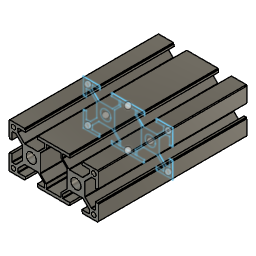
Aluminium extrusion 6030 v2 (Autodesk Fusion 360 design; units mm, degrees)
Autodesk Fusion 360 part; units mm, degrees
sketch "Sketch1" plane through (0, 0, 0) normal (0, 1, 0) x (1, 0, 0)
  circle A0 centre (15, 0) radius 3.4
  line L0 (9, -6) -> (9, 6)
  line L1 (28, -4) -> (28, -9)
  line L2 (28, -9) -> (25.4142, -9)
  line L3 (19, -13) -> (24, -13)
  line L4 (24, -13) -> (24, -10.4142)
  line L5 (25.4142, -9) -> (21, -4.5858)
  line L6 (24, -10.4142) -> (19.5858, -6)
  line L7 (28, 4) -> (28, 9)
  line L8 (28, 9) -> (25.4142, 9)
  line L9 (19, 13) -> (24, 13)
  line L10 (24, 13) -> (24, 10.4142)
  line L11 (24, 10.4142) -> (19.5858, 6)
  line L12 (25.4142, 9) -> (21, 4.5858)
  line L13 (11, -13) -> (6, -13)
  line L14 (6, -13) -> (6, -10.4142)
  line L15 (11, 13) -> (6, 13)
  line L16 (6, 13) -> (6, 10.4142)
  line L17 (6, 10.4142) -> (10.4142, 6)
  line L18 (6, -10.4142) -> (10.4142, -6)
  line L19 (0, -13) -> (5, -13)
  line L20 (5, -13) -> (5, -10)
  line L21 (5, -10) -> (9, -6)
  line L22 (9, 6) -> (5, 10)
  line L23 (5, 10) -> (5, 13)
  line L24 (5, 13) -> (0, 13)
  line L25 (10.4142, -6) -> (19.5858, -6)
  line L26 (10.4142, 6) -> (19.5858, 6)
  line L27 (21, 4.5858) -> (21, -4.5858)
  line L28 (10.5, -15) -> (10.5, -14.5)
  line L29 (10.5, -14.5) -> (11, -14.5)
  line L30 (19.5, -15) -> (19.5, -14.5)
  line L31 (19.5, -14.5) -> (19, -14.5)
  line L32 (30, -4.5) -> (29.5, -4.5)
  line L33 (29.5, -4.5) -> (29.5, -4)
  line L34 (29.5, 4) -> (29.5, 4.5)
  line L35 (29.5, 4.5) -> (30, 4.5)
  line L36 (19.5, 15) -> (19.5, 14.5)
  line L37 (19.5, 14.5) -> (19, 14.5)
  line L38 (11, 14.5) -> (10.5, 14.5)
  line L39 (10.5, 14.5) -> (10.5, 15)
  line L40 (19.5, 15) -> (30, 15)
  line L41 (30, 4.5) -> (30, 15)
  line L42 (19, 13) -> (19, 14.5)
  line L43 (28, 4) -> (29.5, 4)
  line L44 (11, 13) -> (11, 14.5)
  line L45 (29.5, -4) -> (28, -4)
  line L46 (30, -4.5) -> (30, -15)
  line L47 (19.5, -15) -> (30, -15)
  line L48 (19, -14.5) -> (19, -13)
  line L49 (11, -14.5) -> (11, -13)
  circle A1 centre (27, -12) radius 1.5
  circle A2 centre (27, 12) radius 1.5
  line L50 (-28, 4) -> (-28, 9)
  line L51 (-19.5, 15) -> (-30, 15)
  line L52 (-28, 9) -> (-25.4142, 9)
  line L53 (-19, 13) -> (-24, 13)
  line L54 (-5, 13) -> (0, 13)
  line L55 (0, -13) -> (-5, -13)
  line L56 (-29.5, -4) -> (-28, -4)
  line L57 (-19, -13) -> (-24, -13)
  line L58 (-29.5, -4.5) -> (-29.5, -4)
  line L59 (-19.5, -15) -> (-30, -15)
  circle A3 centre (-27, -12) radius 1.5
  circle A4 centre (-27, 12) radius 1.5
  line L60 (-5, 10) -> (-5, 13)
  line L61 (-28, -4) -> (-28, -9)
  line L62 (-6, -13) -> (-6, -10.4142)
  line L63 (-28, -9) -> (-25.4142, -9)
  line L64 (-30, 4.5) -> (-30, 15)
  line L65 (-30, -4.5) -> (-29.5, -4.5)
  line L66 (-29.5, 4.5) -> (-30, 4.5)
  line L67 (-30, -4.5) -> (-30, -15)
  line L68 (-10.4142, -6) -> (-19.5858, -6)
  line L69 (-10.5, -14.5) -> (-11, -14.5)
  line L70 (-19.5, -15) -> (-19.5, -14.5)
  line L71 (-11, -14.5) -> (-11, -13)
  line L72 (-6, 10.4142) -> (-10.4142, 6)
  line L73 (-19.5, -14.5) -> (-19, -14.5)
  line L74 (-10.5, -15) -> (-10.5, -14.5)
  line L75 (-11, 13) -> (-11, 14.5)
  line L76 (-10.5, 14.5) -> (-10.5, 15)
  line L77 (-28, 4) -> (-29.5, 4)
  line L78 (-6, 13) -> (-6, 10.4142)
  line L79 (-11, 14.5) -> (-10.5, 14.5)
  line L80 (-24, -13) -> (-24, -10.4142)
  line L81 (-5, -13) -> (-5, -10)
  line L82 (-6, -10.4142) -> (-10.4142, -6)
  line L83 (-11, -13) -> (-6, -13)
  line L84 (-19.5, 14.5) -> (-19, 14.5)
  line L85 (-19, -14.5) -> (-19, -13)
  line L86 (-24, 13) -> (-24, 10.4142)
  line L87 (-5, -10) -> (-9, -6)
  line L88 (-29.5, 4) -> (-29.5, 4.5)
  line L89 (-11, 13) -> (-6, 13)
  line L90 (-24, 10.4142) -> (-19.5858, 6)
  line L91 (-10.4142, 6) -> (-19.5858, 6)
  line L92 (-21, 4.5858) -> (-21, -4.5858)
  circle A5 centre (-15, 0) radius 3.4
  line L93 (-9, -6) -> (-9, 6)
  line L94 (-9, 6) -> (-5, 10)
  line L95 (-24, -10.4142) -> (-19.5858, -6)
  line L96 (-19.5, 15) -> (-19.5, 14.5)
  line L97 (-19, 13) -> (-19, 14.5)
  line L98 (-25.4142, -9) -> (-21, -4.5858)
  line L99 (-25.4142, 9) -> (-21, 4.5858)
  line L100 (-10.5, 15) -> (0, 15)
  line L101 (0, 15) -> (10.5, 15)
  line L102 (-10.5, -15) -> (0, -15)
  line L103 (0, -15) -> (10.5, -15)
  dimension "d4" = 6.8
  dimension "d19" = 8
  dimension "d20" = 30
  dimension "d21" = 3
  dimension "d22" = 12
  dimension "d35" = 18
  dimension "d36" = 7
  dimension "d37" = 2
  constraint vertical L0
  constraint perpendicular L1 L2
  constraint perpendicular L3 L4
  constraint perpendicular L7 L8
  constraint perpendicular L9 L10
  constraint perpendicular L13 L14
  constraint perpendicular L17 L18
  constraint perpendicular L19 L20
  constraint parallel L20 L23
  constraint perpendicular L23 L24
  constraint horizontal L25
  constraint horizontal L26
  constraint perpendicular L26 L27
  constraint perpendicular L36 L40
  constraint perpendicular L40 L41
  constraint perpendicular L37 L42
  constraint perpendicular L34 L43
  constraint perpendicular L38 L44
  constraint perpendicular L33 L45
  constraint perpendicular L46 L47
  constraint perpendicular L31 L48
  constraint perpendicular L13 L49
  constraint perpendicular L76 L100
  constraint perpendicular L74 L102
  measures "d4" diameter of A0
  measures "d19" distance of L43 L45
  measures "d20" distance of L40 L47
  measures "d21" diameter of A1
  measures "d22" distance of L0 L27
  measures "d35" distance of L4 L14
  measures "d36" distance of L3 L25
  measures "d37" distance of L1 L46
extrude "Extrude1" add sketch "Sketch1" along normal mid plane 100
fillet "Fillet1" radius 0.5 4 edges at (-30, 0, 15) (30, 0, 15) (30, 0, -15) (-30, 0, -15)
fillet "Fillet2" radius 0.3 16 edges at (-24, 0, 13) (-28, 0, 9) (-5, 0, 13) (6, 0, 13) (-6, 0, 13) (24, 0, 13) (28, 0, 9) (5, 0, 13) (-28, 0, -9) (-24, 0, -13) (-5, 0, -13) (6, 0, -13) (-6, 0, -13) (5, 0, -13) (24, 0, -13) (28, 0, -9)
fillet "Fillet3" radius 0.5 8 edges at (5, 0, -10) (-5, 0, -10) (-5, 0, 10) (5, 0, 10) (6, 0, 10.4142) (-6, 0, 10.4142) (-6, 0, -10.4142) (6, 0, -10.4142)
fillet "Fillet4" radius 0.5 16 edges at (-10.4142, 0, -6) (19.5858, 0, -6) (10.4142, 0, -6) (-19.5858, 0, -6) (-9, 0, -6) (-9, 0, 6) (21, 0, 4.5858) (21, 0, -4.5858) (9, 0, -6) (9, 0, 6) (-21, 0, 4.5858) (-21, 0, -4.5858) (-10.4142, 0, 6) (19.5858, 0, 6) (10.4142, 0, 6) (-19.5858, 0, 6)
fillet "Fillet5" radius 0.3 8 edges at (24, 0, 10.4142) (25.4142, 0, 9) (25.4142, 0, -9) (-25.4142, 0, -9) (24, 0, -10.4142) (-24, 0, -10.4142) (-24, 0, 10.4142) (-25.4142, 0, 9)
